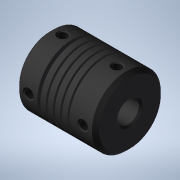
# Autodesk Inventor part: E60063
Saved by Autodesk Inventor 2021 (Build 250183000, 183)
## iProperties
Category: PARTsolutions
Company: IFMELECTRONIC
Created: 2026-05-26
Part Number: E60063
Material: Generic
Catalog Web Link: www.3dfindit.com
Description: E60063-Couplings for encoders
Vendor: IFMELECTRONIC
Document SubType Name: Modeling
Designer: psAdmin
Manufacturer: IFMELECTRONIC
Mass: 4.76615 g
Surface Area: 49.677 cm^2
Volume: 4.76615 cm^3
Density: 1 g/cm^3
Appearance: PSOLRGB-176-176-176
PSOL_IDENT_0: {$CADENAS_DATA/23d-libs/ifm_electronic/_cat_/de/cf/e60063.prj},152 {VTYP=3D},{NB=E60063},{LINA=E6006
PSOL_IDENT_1: 3},{NN=E60063},{DATE=30.03.2026 08:41:04},{GEOMDATE=27.03.2026 14:39:40},{VERSION=},{LINEID=10},{WBV
PSOL_IDENT_2: AR=},{WBNUMERIC=}  {NB=E60063},{LINA=E60063},{KT=DUMMY},{PREVIEW=../../../_pool_/e0/21/pc_e60063aa_0
PSOL_IDENT_3: 1.png},{PRODUKTFOTO=../../../_pool_/e0/21/pc_e60063aa_01.png},{DESCRIPTIONSHORT=E60063: Wendelkupplu
PSOL_IDENT_4: ng für Drehgeber; Ø 19 / L = 22 mm},{DESCLONG=Wendelkupplung für Drehgeber; Ø 19 / L = 22 mm},{BN=E6
PSOL_IDENT_5: 0063},{MANUNAME=ifm electronic gmbh},{DATASHEET=DATASHEET},{MANUTYPEDESC=COUPLING 19,2-6-6-22-SV},{E
PSOL_IDENT_6: RPGRSUPPLIER=DN},{DELTIME=2.0},{ARTICLE_STATUS=false},{ORDERUNIT=PCE},{CONTENTUNIT=},{NOCUPEROU=1},{
PSOL_IDENT_7: PRICEQUANTITY=1},{QUANTITYMIN=1},{QUANTITYINT=1},{DATASHEET_DEU=https://www.ifm.com/de/de/product/E6
PSOL_IDENT_8: 0063},{DATASHEET_ENG=https://www.ifm.com/de/en/product/E60063},{DATASHEET_=https://www.ifm.com/de/en
PSOL_IDENT_9: /product/E60063},{DATASHEET_FRA=https://www.ifm.com/fr/fr/product/E60063}
NB: E60063
NN: E60063
NT: Kupplungen für Drehgeber
NBSYN: $BN.
LINA: E60063
CATALOG: ifm electronic
PREVIEW: ../../../_pool_/e0/21/pc_e60063aa_01.png
PRODUKTFOTO: ../../../_pool_/e0/21/pc_e60063aa_01.png
DESCRIPTIONSHORT: E60063: Wendelkupplung für Drehgeber; Ø 19 / L = 22 mm
DESCLONG: Wendelkupplung für Drehgeber; Ø 19 / L = 22 mm
BN: E60063
MANUNAME: ifm electronic gmbh
DATASHEET: DATASHEET
SUPPLIER: IFMELECTRONIC
ARTICLENO: E60063
BOMINFO: E60063
CREATOR: CADENAS GmbH
Title: E60063
Author: Cadenas PARTsolutions
Comments: Couplings for encoders
Autodesk Inventor part; units mm, degrees
ref_plane "YZ Plane" through (0, 0, 0) normal (1, 0, 0) x (0, 1, 0)
ref_plane "XZ Plane" through (0, 0, 0) normal (0, 1, 0) x (-1, 0, 0)
ref_plane "XY Plane" through (0, 0, 0) normal (0, 0, 1) x (1, 0, 0)
sketch "Sketch_1" plane through (0, 0, 0) normal (0, 0, 1) x (1, 0, 0)
  line L0 (22, 0) -> (0, 0)
  line L1 (0, 3.5) -> (0.5, 3)
  line L2 (0.5, 3) -> (21.5, 3)
  line L3 (21.5, 3) -> (22, 3.5)
  line L4 (22, 3.5) -> (22, 8.5)
  line L5 (22, 8.5) -> (21, 9.5)
  line L6 (21, 9.5) -> (1, 9.5)
  line L7 (1, 9.5) -> (0, 8.5)
  line L8 (0, 8.5) -> (0, 3.5)
  constraints: 18 end point
revolve "Revolution1" add sketch "Sketch_1" angle 360 about axis through (22, 0, 0) along (1, 0, 0)
sketch "Sketch_2" plane through (0, 0, 0) normal (0, -0.7071068, 0.7071068) x (1, 0, 0)
  line L0 (6, 20) -> (6, -9.0286)
  line L1 (6, -9.0286) -> (6.9157, 9.5)
  line L2 (6.9157, 9.5) -> (8.4175, 9.5)
  line L3 (8.4175, 9.5) -> (7.4796, -9.4768)
  line L4 (7.4796, -9.4768) -> (7.9778, -9.4768)
  line L5 (7.9778, -9.4768) -> (8.9157, 9.5)
  line L6 (8.9157, 9.5) -> (10.4175, 9.5)
  line L7 (10.4175, 9.5) -> (9.4796, -9.4768)
  line L8 (9.4796, -9.4768) -> (9.9778, -9.4768)
  line L9 (9.9778, -9.4768) -> (10.9157, 9.5)
  line L10 (10.9157, 9.5) -> (12.4175, 9.5)
  line L11 (12.4175, 9.5) -> (11.4796, -9.4768)
  line L12 (11.4796, -9.4768) -> (11.9778, -9.4768)
  line L13 (11.9778, -9.4768) -> (12.9157, 9.5)
  line L14 (12.9157, 9.5) -> (14.4175, 9.5)
  line L15 (14.4175, 9.5) -> (13.4796, -9.4768)
  line L16 (13.4796, -9.4768) -> (13.9778, -9.4768)
  line L17 (13.9778, -9.4768) -> (15.4346, 20)
  line L18 (15.4346, 20) -> (6, 20)
  constraints: 38 end point
extrude "Extrusion1" cut sketch "Sketch_2" along normal mid plane 40
sketch "Sketch_3" plane through (0, 0, 0) normal (0, -0.7071068, 0.7071068) x (1, 0, 0)
  line L0 (15.3, -12.5) -> (16, -12.5)
  line L1 (16, -12.5) -> (16, 1.6701)
  line L2 (16, 1.6701) -> (15.3, -12.5)
  constraints: 6 end point
extrude "Extrusion2" cut sketch "Sketch_3" along normal mid plane 40
sketch "Sketch_4" plane through (0, 0, 0) normal (0, 0, 1) x (1, 0, 0)
  line L0 (3.5, 2) -> (3.5, 9.5)
  line L1 (3.5, 9.5) -> (5, 9.5)
  line L2 (5, 9.5) -> (4.7295, 9.2295)
  line L3 (4.7295, 9.2295) -> (4.7295, 2)
  line L4 (4.7295, 2) -> (3.5, 2)
  line L5 (3.5, 2) -> (3.5, 9.5)
  constraints: 12 end point
revolve "Revolution2" cut sketch "Sketch_4" angle 360 about axis through (3.5, 2, 0) along (0, -1, 0)
thread "Thread1" size "M3x0.5" class "6H" standard "ISO Metric profile" length 7.2295
sketch "Sketch_5" plane through (0, 0, 0) normal (0, 0, 1) x (1, 0, 0)
  line L0 (18.5, 2) -> (18.5, 9.5)
  line L1 (18.5, 9.5) -> (20, 9.5)
  line L2 (20, 9.5) -> (19.7295, 9.2295)
  line L3 (19.7295, 9.2295) -> (19.7295, 2)
  line L4 (19.7295, 2) -> (18.5, 2)
  line L5 (18.5, 2) -> (18.5, 9.5)
  constraints: 12 end point
revolve "Revolution3" cut sketch "Sketch_5" angle 360 about axis through (18.5, 2, 0) along (0, -1, 0)
thread "Thread2" size "M3x0.5" class "6H" standard "ISO Metric profile" length 7.2295
sketch "Sketch_6" plane through (0, 0, 0) normal (0, 1, 0) x (-1, 0, 0)
  line L0 (-3.5, 9.5) -> (-3.5, 2)
  line L1 (-3.5, 2) -> (-4.7295, 2)
  line L2 (-4.7295, 2) -> (-4.7295, 9.2295)
  line L3 (-4.7295, 9.2295) -> (-5, 9.5)
  line L4 (-5, 9.5) -> (-3.5, 9.5)
  line L5 (-3.5, 9.5) -> (-3.5, 2)
  constraints: 12 end point
revolve "Revolution4" cut sketch "Sketch_6" angle 360 about axis through (3.5, 0, 9.5) along (0, 0, 1)
thread "Thread3" size "M3x0.5" class "6H" standard "ISO Metric profile" length 7.2295
sketch "Sketch_7" plane through (0, 0, 0) normal (0, 1, 0) x (-1, 0, 0)
  line L0 (-18.5, 9.5) -> (-18.5, 2)
  line L1 (-18.5, 2) -> (-19.7295, 2)
  line L2 (-19.7295, 2) -> (-19.7295, 9.2295)
  line L3 (-19.7295, 9.2295) -> (-20, 9.5)
  line L4 (-20, 9.5) -> (-18.5, 9.5)
  line L5 (-18.5, 9.5) -> (-18.5, 2)
  constraints: 12 end point
revolve "Revolution5" cut sketch "Sketch_7" angle 360 about axis through (18.5, 0, 9.5) along (0, 0, 1)
thread "Thread4" size "M3x0.5" class "6H" standard "ISO Metric profile" length 7.2295
body "Solid1"
